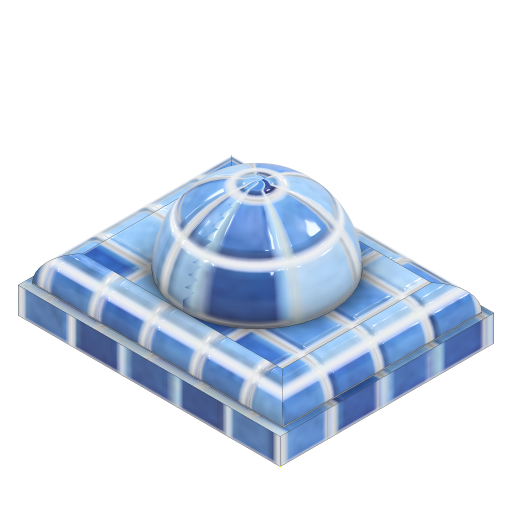
# Autodesk Inventor part: che
Saved by Autodesk Inventor 2024.3 (Build 283343000, 343)
## iProperties
Created: 2025-09-02
Part Number: che
Material: Generic
Document SubType Name: Modeling
Designer: danie
Density: 1 g/cm^3
Appearance: 1in Squares - Mosaic Blue
Author: danie
Autodesk Inventor part; units mm, degrees
ref_plane "YZ Plane" through (0, 0, 0) normal (1, 0, 0) x (0, 1, 0)
ref_plane "XZ Plane" through (0, 0, 0) normal (0, 1, 0) x (-1, 0, 0)
ref_plane "XY Plane" through (0, 0, 0) normal (0, 0, 1) x (1, 0, 0)
sketch "Sketch1" plane through (0, 0, 0) normal (0, 1, 0) x (-1, 0, 0)
  line L0 (0, 0) -> (130, 0)
  line L1 (130, 0) -> (130, -106)
  line L2 (130, -106) -> (0, -106)
  line L3 (0, -106) -> (0, 0)
  line L4 (130, 0) -> (130, -3)
  line L5 (127, -4.0545) -> (0, -4.0545)
  line L6 (0, -4.0545) -> (3, -4.0545)
  line L7 (3, -4.0545) -> (3, -106)
  line L8 (3, -106) -> (3, -103)
  line L9 (3, -103) -> (3, -101.9174)
  line L10 (3, -103) -> (130, -103)
  line L11 (130, -3) -> (127, -4.0545)
  line L12 (130, -103) -> (127, -103)
  line L13 (127, -103) -> (127, -4.0545)
  line L14 (127, -4.0545) -> (0, -4.0545)
  line L15 (0, 0) -> (0, -106)
  line L16 (0, -106) -> (130, -106)
  line L17 (130, -106) -> (130, 0)
  line L18 (127, -4.0545) -> (127, -103)
  line L19 (127, -103) -> (3, -103)
  line L20 (3, -103) -> (3, -4.0545)
  line L21 (3, -4.0545) -> (127, -4.0545)
  dimension "d0" = 130
  dimension "d1" = 106
  dimension "d2" = 3
  dimension "d3" = 3
  dimension "d4" = 3
  dimension "d5" = 3
  constraints: 44 end point, 7 point on line, 6 collinear, 6 perpendicular, 3 parallel, 1 horizontal
  measures "d0" distance of L1.end L2.end
  measures "d1" distance of L0.end L1.end
  measures "d2" distance of L0.end L4.end
  measures "d3" distance of L5.end L6.end
  measures "d4" distance of L7.end L8.end
  measures "d5" distance of L10.end L12.end
sketch "Sketch2" plane through (0, 0, 0) normal (0, 1, 0) x (-1, 0, 0)
  point P0 (0, 0)
extrude "Extrusion1" add sketch "Sketch1" along normal blind 13 contours L0 L1 L11 L5 L3 | L5 L7 L2 L3 | L1 L10 L13 L11 | L1 L2 L7 L10
sketch "Sketch3" plane through (0, 13, 0) normal (0, 1, 0) x (1, 0, 0)
  line L0 (-130, 106) -> (-130, 0) projected
  line L1 (0, 106) -> (-130, 106) projected
  line L2 (-130, 106) -> (0, 106)
  line L3 (0, 106) -> (0, 0)
  line L4 (0, 0) -> (-130, 0)
  line L5 (-130, 106) -> (-130, 0)
  line L6 (-3, 4.0545) -> (-127, 4.0545) projected
  line L7 (-3, 103) -> (-3, 4.0545) projected
  line L8 (-127, 4.0545) -> (-3, 4.0545)
  line L9 (-3, 4.0545) -> (-3, 103)
  line L10 (-3, 103) -> (-127, 103)
  line L11 (-127, 103) -> (-127, 4.0545)
  constraints: 16 end point, 5 perpendicular, 2 collinear, 1 horizontal
extrude "Extrusion2" add sketch "Sketch3" along normal blind 13 contours L6 L11 L10 L7
fillet "Fillet1" radius 12.5 4 edges at (-65, 26, -103) (-127, 26, -53.5272) (-65, 26, -4.0545) (-3, 26, -53.5272)
sketch "Sketch4" plane through (0, 26, 0) normal (0, 1, 0) x (1, 0, 0)
  line L0 (-114.5, 16.5545) -> (-114.5, 90.5) projected
  line L1 (-114.5, 90.5) -> (-15.5, 90.5) projected
  line L2 (-114.5, 90.5) -> (-15.5, 90.5)
  line L3 (-15.5, 90.5) -> (-65, 90.5)
  line L4 (-15.5, 90.5) -> (-65, 90.5)
  line L5 (-114.5, 16.5545) -> (-114.5, 90.5)
  line L6 (-114.5, 90.5) -> (-114.5, 53.5272)
  circle A0 centre (-65, 53.5272) radius 36.9728
  line L7 (-101.9728, 53.5272) -> (-28.0272, 53.5272)
  point P0 (0, 0)
  constraints: 12 end point, 3 collinear, 3 point on circle, 2 midpoint, 1 centre point, 1 horizontal
revolve "Revolution1" add sketch "Sketch4" angle 180 about axis through (-101.9728, 26, -53.5272) along (1, 0, 0) picked at (-57.3159, 68.6475) contours L7 A0
sketch "Sketch5" plane through (0, 13, 0) normal (0, -1, 0) x (1, 0, 0)
  line L0 (0, 0) -> (0, -106) projected
  line L1 (0, -57.157) -> (-67.076, -57.157)
  line L2 (-67.076, -57.157) -> (-130, -57.157)
  line L3 (-130, -106) -> (-130, 0) projected
  arc A0 (-65, -90.5) -> (-65, -16.5545) centre (-65, -53.5272) ccw projected
  circle A1 centre (-65.5426, -54.6499) radius 1.2469
  circle A2 centre (-65, -53.5272) radius 35
  point P0 (-99.8113, -57.157)
  point P1 (-30.1887, -57.157)
  dimension "d12" = 70
  constraints: 4 end point, 3 point on line, 1 centre point, 1 coincident, 1 horizontal, 3 other
  measures "d12" diameter of A2
revolve "Revolution2" cut sketch "Sketch5" angle 180 about axis through (0, 13, -57.157) along (1, 0, 0) picked at (-43.0495, -59.7228) contours A2 L2 L1
body "Solid1"
